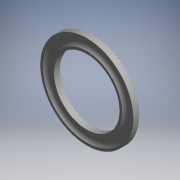
# Autodesk Inventor part: 51111 Shaft raceway disc
Saved by Autodesk Inventor 2023 (Build 270158000, 158)
## iProperties
Part Number: 51111 Shaft raceway disc
Material: 一般
Catalog Web Link: www.cadenas.de
Description: tb sdt srd-
Vendor: NTN
Document SubType Name: Modeling
Designer: partserver
Manufacturer: NTN
Mass: 10.8737 g
Surface Area: 71.6865 cm^2
Volume: 10.8737 cm^3
Density: 1 g/cm^3
Appearance: PSOLRGB-192-192-192
Category: PARTsolutions
Company: NTN
PSOL_IDENT_0: {$CADENAS_DATA\23d-libs\ntn\ball_roller_bearings\thrust_b\tb_sdt_or.prj},195 {VTYP=3D},{NB=51111 Sha
PSOL_IDENT_1: ft raceway disc},{LINA=51111 Shaft raceway disc},{NN=tb sdt srd},{DATE=21.12.2021 04:23:12},{GEOMDAT
PSOL_IDENT_2: E=08.04.2020 13:28:19},{VERSION=},{LINEID=11140},{WBVAR=},{WBNUMERIC=}  {NB=51111 Shaft raceway disc
PSOL_IDENT_3: },{LINA=51111 Shaft raceway disc},{KT=DUMMY},{IDNR=},{SD=55},{D=78},{T=16},{R=0.6},{ORDER=51111},{CA=
PSOL_IDENT_4: 35},{COA=93},{CAF=3 550},{COAF=9 500},{NG=2 800},{NO=4 000},{D1=78},{SD1=57},{MASS=0.23},{DA1=69},{D
PSOL_IDENT_5: A=64},{RAS=0,6},{X=10.50000},{BN=14},{X1=11.50000},{O=208.81000},{T1=5.33333},{T2=5.33333},{RB=4.480
PSOL_IDENT_6: 00},{BN1=13.00000}
NB: 51111 Shaft raceway disc
NN: tb sdt srd
NBSYN: $ORDER. Shaft raceway disc
LINA: 51111 Shaft raceway disc
CATALOG: NTN Corporation
SD: 55
D: 78
T: 16
R: 0.6
ORDER: 51111
CA: 35
COA: 93
CAF: 3 550
COAF: 9 500
NG: 2 800
NO: 4 000
D1: 78
SD1: 57
MASS: 0.23
DA1: 69
DA: 64
RAS: 0,6
SUPPLIER: NTN
ARTICLENO: 51111 Shaft raceway disc
BOMINFO: 51111 Shaft raceway disc
CREATOR: CADENAS GmbH
Title: 51111 Shaft raceway disc
Author: Cadenas PARTsolutions
Autodesk Inventor part; units mm, degrees
sketch "Sketch_1" plane through (0, 0, 0) normal (0, 0, 1) x (1, 0, 0)
  line L0 (0, 16) -> (0, 10.6667)
  line L1 (-39, 10.6667) -> (-36.8499, 10.6667)
  arc A0 (-29.6501, 10.6667) -> (-36.8499, 10.6667) centre (-33.25, 8) ccw
  line L2 (-29.6501, 10.6667) -> (-27.5, 10.6667)
  line L3 (-27.5, 10.6667) -> (-27.5, 15.4)
  arc A1 (-27.5, 15.4) -> (-28.1, 16) centre (-28.1, 15.4) ccw
  line L4 (-28.1, 16) -> (-38.4, 16)
  arc A2 (-38.4, 16) -> (-39, 15.4) centre (-38.4, 15.4) ccw
  line L5 (-39, 15.4) -> (-39, 10.6667)
  constraints: 12 end point, 6 point on circle, 3 centre point
revolve "Revolution1" add sketch "Sketch_1" angle 360 about axis through (0, 16, 0) along (0, 1, 0)
ref_plane "tb_sdt_srd_XY" through (0, 0, 0) normal (0, 1, 0) x (1, 0, 0)
ref_plane "tb_sdt_srd_YZ" through (0, 0, 0) normal (1, 0, 0) x (0, 0, -1)
ref_plane "tb_sdt_srd_ZX" through (0, 0, 0) normal (0, 0, -1) x (0, 1, 0)
ref_plane "tb_sdt_srd1_1_XY" through (0, 8, -33.25) normal (0, 1, 0) x (1, 0, 0)
ref_plane "tb_sdt_srd1_1_YZ" through (0, 8, -33.25) normal (1, 0, 0) x (0, 0, -1)
ref_plane "tb_sdt_srd1_1_ZX" through (0, 8, -33.25) normal (0, 0, -1) x (0, 1, 0)
ref_plane "tb_sdt_srd1_10_XY" through (25.9959, 8, 20.731) normal (0, 1, 0) x (1, 0, 0)
ref_plane "tb_sdt_srd1_10_YZ" through (25.9959, 8, 20.731) normal (1, 0, 0) x (0, 0, -1)
ref_plane "tb_sdt_srd1_10_ZX" through (25.9959, 8, 20.731) normal (0, 0, -1) x (0, 1, 0)
ref_plane "tb_sdt_srd1_11_XY" through (32.4164, 8, 7.3988) normal (0, 1, 0) x (1, 0, 0)
ref_plane "tb_sdt_srd1_11_YZ" through (32.4164, 8, 7.3988) normal (1, 0, 0) x (0, 0, -1)
ref_plane "tb_sdt_srd1_11_ZX" through (32.4164, 8, 7.3988) normal (0, 0, -1) x (0, 1, 0)
ref_plane "tb_sdt_srd1_12_XY" through (32.4164, 8, -7.3988) normal (0, 1, 0) x (1, 0, 0)
ref_plane "tb_sdt_srd1_12_YZ" through (32.4164, 8, -7.3988) normal (1, 0, 0) x (0, 0, -1)
ref_plane "tb_sdt_srd1_12_ZX" through (32.4164, 8, -7.3988) normal (0, 0, -1) x (0, 1, 0)
ref_plane "tb_sdt_srd1_13_XY" through (25.9959, 8, -20.731) normal (0, 1, 0) x (1, 0, 0)
ref_plane "tb_sdt_srd1_13_YZ" through (25.9959, 8, -20.731) normal (1, 0, 0) x (0, 0, -1)
ref_plane "tb_sdt_srd1_13_ZX" through (25.9959, 8, -20.731) normal (0, 0, -1) x (0, 1, 0)
ref_plane "tb_sdt_srd1_14_XY" through (14.4266, 8, -29.9572) normal (0, 1, 0) x (1, 0, 0)
ref_plane "tb_sdt_srd1_14_YZ" through (14.4266, 8, -29.9572) normal (1, 0, 0) x (0, 0, -1)
ref_plane "tb_sdt_srd1_14_ZX" through (14.4266, 8, -29.9572) normal (0, 0, -1) x (0, 1, 0)
ref_plane "tb_sdt_srd1_2_XY" through (-14.4266, 8, -29.9572) normal (0, 1, 0) x (1, 0, 0)
ref_plane "tb_sdt_srd1_2_YZ" through (-14.4266, 8, -29.9572) normal (1, 0, 0) x (0, 0, -1)
ref_plane "tb_sdt_srd1_2_ZX" through (-14.4266, 8, -29.9572) normal (0, 0, -1) x (0, 1, 0)
ref_plane "tb_sdt_srd1_3_XY" through (-25.9959, 8, -20.731) normal (0, 1, 0) x (1, 0, 0)
ref_plane "tb_sdt_srd1_3_YZ" through (-25.9959, 8, -20.731) normal (1, 0, 0) x (0, 0, -1)
ref_plane "tb_sdt_srd1_3_ZX" through (-25.9959, 8, -20.731) normal (0, 0, -1) x (0, 1, 0)
ref_plane "tb_sdt_srd1_4_XY" through (-32.4164, 8, -7.3988) normal (0, 1, 0) x (1, 0, 0)
ref_plane "tb_sdt_srd1_4_YZ" through (-32.4164, 8, -7.3988) normal (1, 0, 0) x (0, 0, -1)
ref_plane "tb_sdt_srd1_4_ZX" through (-32.4164, 8, -7.3988) normal (0, 0, -1) x (0, 1, 0)
ref_plane "tb_sdt_srd1_5_XY" through (-32.4164, 8, 7.3988) normal (0, 1, 0) x (1, 0, 0)
ref_plane "tb_sdt_srd1_5_YZ" through (-32.4164, 8, 7.3988) normal (1, 0, 0) x (0, 0, -1)
ref_plane "tb_sdt_srd1_5_ZX" through (-32.4164, 8, 7.3988) normal (0, 0, -1) x (0, 1, 0)
ref_plane "tb_sdt_srd1_6_XY" through (-25.9959, 8, 20.731) normal (0, 1, 0) x (1, 0, 0)
ref_plane "tb_sdt_srd1_6_YZ" through (-25.9959, 8, 20.731) normal (1, 0, 0) x (0, 0, -1)
ref_plane "tb_sdt_srd1_6_ZX" through (-25.9959, 8, 20.731) normal (0, 0, -1) x (0, 1, 0)
ref_plane "tb_sdt_srd1_7_XY" through (-14.4266, 8, 29.9572) normal (0, 1, 0) x (1, 0, 0)
ref_plane "tb_sdt_srd1_7_YZ" through (-14.4266, 8, 29.9572) normal (1, 0, 0) x (0, 0, -1)
ref_plane "tb_sdt_srd1_7_ZX" through (-14.4266, 8, 29.9572) normal (0, 0, -1) x (0, 1, 0)
ref_plane "tb_sdt_srd1_8_XY" through (0, 8, 33.25) normal (0, 1, 0) x (1, 0, 0)
ref_plane "tb_sdt_srd1_8_YZ" through (0, 8, 33.25) normal (1, 0, 0) x (0, 0, -1)
ref_plane "tb_sdt_srd1_8_ZX" through (0, 8, 33.25) normal (0, 0, -1) x (0, 1, 0)
ref_plane "tb_sdt_srd1_9_XY" through (14.4266, 8, 29.9572) normal (0, 1, 0) x (1, 0, 0)
ref_plane "tb_sdt_srd1_9_YZ" through (14.4266, 8, 29.9572) normal (1, 0, 0) x (0, 0, -1)
ref_plane "tb_sdt_srd1_9_ZX" through (14.4266, 8, 29.9572) normal (0, 0, -1) x (0, 1, 0)
body "Solid1"
